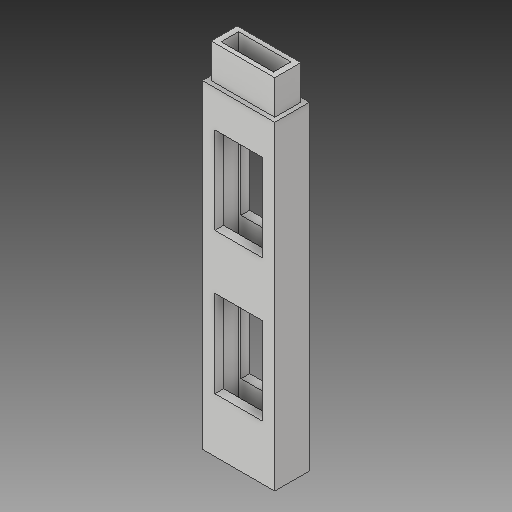
# Autodesk Inventor part: Pizza2
Saved by Autodesk Inventor 2018 (Build 220112000, 112)
## iProperties
Created: 2018-03-29
Part Number: Pizza2
Material: Generic
Document SubType Name: Modeling
Designer: MIABo
Density: 1 g/cm^3
Appearance: Default
Mass: 10.3912 g
Surface Area: 86.8088 cm^2
Volume: 10.3912 cm^3
Author: MIABo
## iProperties of the stored document Pizza2_3DPrint.ipt
Created: 2018-03-29
Part Number: Pizza2_3DPrint
Material: Generic
Document SubType Name: Modeling
Designer: MIABo
Density: 1 g/cm^3
Appearance: Default
Author: MIABo
Autodesk Inventor part; units mm, degrees
ref_plane "YZ Plane" through (0, 0, 0) normal (1, 0, 0) x (0, 1, 0)
ref_plane "XZ Plane" through (0, 0, 0) normal (0, 1, 0) x (-1, 0, 0)
ref_plane "XY Plane" through (0, 0, 0) normal (0, 0, 1) x (1, 0, 0)
sketch "Sketch2" plane through (0, 0, 0) normal (0, 1, 0) x (-1, 0, 0)
  line L0 (9.271, 3.81) -> (-9.271, 3.81)
  line L1 (-9.271, 3.81) -> (-9.271, -3.81)
  line L2 (-9.271, -3.81) -> (9.271, -3.81)
  line L3 (9.271, -3.81) -> (9.271, 3.81)
  line L4 (9.271, 3.81) -> (-9.271, -3.81) construction
  line L5 (-9.271, 3.81) -> (9.271, -3.81) construction
  point P0 (0, 0)
  dimension "d3" = 18.542
  dimension "d4" = 7.62
  constraints: 12 end point, 2 midpoint, 2 parallel, 1 horizontal, 1 perpendicular
  measures "d3" distance of L2.end L1.end
  measures "d4" distance of L1.end L0.end
extrude "Extrusion2" add sketch "Sketch2" along normal blind 114.3
sketch "Sketch3" plane through (0, 114.3, 0) normal (0, 1, 0) x (1, 0, 0)
  point P0 (0, 0)
sketch "Sketch4" plane through (0, 0, 0) normal (0, -1, 0) x (1, 0, 0)
  line L0 (-10.541, -5.08) -> (10.541, -5.08)
  line L1 (10.541, -5.08) -> (10.541, 5.08)
  line L2 (10.541, 5.08) -> (-10.541, 5.08)
  line L3 (-10.541, 5.08) -> (-10.541, -5.08)
  line L4 (-10.541, -5.08) -> (10.541, 5.08) construction
  line L5 (10.541, -5.08) -> (-10.541, 5.08) construction
  point P0 (0, 0)
  dimension "d7" = 21.082
  dimension "d8" = 10.16
  constraints: 12 end point, 2 midpoint, 2 parallel, 1 horizontal, 1 perpendicular
  measures "d7" distance of L2.end L1.end
  measures "d8" distance of L1.end L0.end
extrude "Extrusion3" add sketch "Sketch4" against normal blind 93.1926
hole "Hole1" at (0, 114.3, 0) direction (0, -1, 0) diameter 3.302 end through all
sketch "Sketch5" plane through (0, 114.3, 0) normal (0, 1, 0) x (1, 0, 0)
  line L0 (7.62, -2.54) -> (-7.62, -2.54)
  line L1 (-7.62, -2.54) -> (-7.62, 2.54)
  line L2 (-7.62, 2.54) -> (7.62, 2.54)
  line L3 (7.62, 2.54) -> (7.62, -2.54)
  line L4 (7.62, -2.54) -> (-7.62, 2.54) construction
  line L5 (-7.62, -2.54) -> (7.62, 2.54) construction
  point P0 (0, 0)
  dimension "d18" = 15.24
  dimension "d19" = 5.08
  constraints: 12 end point, 2 midpoint, 2 parallel, 1 horizontal, 1 perpendicular
  measures "d18" distance of L1.end L2.end
  measures "d19" distance of L0.end L1.end
extrude "Extrusion4" cut sketch "Sketch5" against normal blind 105.8926
sketch "Sketch6" plane through (0, 114.3, 0) normal (0, 1, 0) x (1, 0, 0)
  line L0 (14.2875, -6.35) -> (-14.2875, -6.35)
  line L1 (-14.2875, -6.35) -> (-14.2875, 6.35)
  line L2 (-14.2875, 6.35) -> (14.2875, 6.35)
  line L3 (14.2875, 6.35) -> (14.2875, -6.35)
  line L4 (14.2875, -6.35) -> (-14.2875, 6.35) construction
  line L5 (-14.2875, -6.35) -> (14.2875, 6.35) construction
  point P0 (0, 0)
  constraints: 12 end point, 2 midpoint, 2 parallel, 1 horizontal, 1 perpendicular
extrude "Extrusion5" cut sketch "Sketch6" against normal blind 11.1125
sketch "Sketch7" plane through (-10.541, 0, 5.08) normal (0, 0, 1) x (1, 0, 0)
  line L0 (3.6195, 82.55) -> (17.4625, 82.55)
  line L1 (17.4625, 82.55) -> (17.4625, 57.15)
  line L2 (17.4625, 57.15) -> (3.6195, 57.15)
  line L3 (3.6195, 57.15) -> (3.6195, 82.55)
  line L4 (3.6195, 82.55) -> (17.4625, 57.15) construction
  line L5 (17.4625, 82.55) -> (3.6195, 57.15) construction
  line L6 (3.6195, 15.875) -> (17.4625, 15.875)
  line L7 (17.4625, 15.875) -> (17.4625, 41.275)
  line L8 (17.4625, 41.275) -> (3.6195, 41.275)
  line L9 (3.6195, 41.275) -> (3.6195, 15.875)
  line L10 (3.6195, 15.875) -> (17.4625, 41.275) construction
  line L11 (17.4625, 15.875) -> (3.6195, 41.275) construction
  point P0 (10.541, 0)
  point P1 (10.541, 69.85)
  point P2 (10.541, 28.575)
  constraints: 24 end point, 4 midpoint, 4 parallel, 2 horizontal, 2 perpendicular, 1 point on line
extrude "Extrusion6" cut sketch "Sketch7" against normal blind 25.4
body "Solid2"
